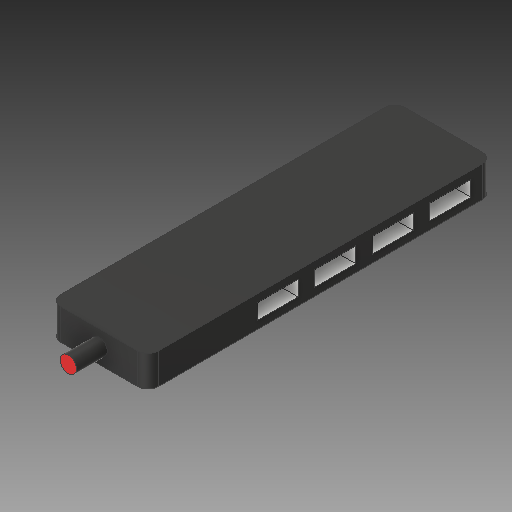
# Autodesk Inventor part: usbHub
Saved by Autodesk Inventor 2018 (Build 220112000, 112)
## iProperties
Created: 2018-08-03
Part Number: usbHub
Material: ABS Plastic
Document SubType Name: Modeling
Designer: Cole Tucker
Density: 1.06 g/cm^3
Appearance: Smooth - White
Mass: 30.4132 g
Surface Area: 110.112 cm^2
Volume: 28.6917 cm^3
Author: Cole Tucker
Autodesk Inventor part; units mm, degrees
ref_plane "YZ Plane" through (0, 0, 0) normal (1, 0, 0) x (0, 1, 0)
ref_plane "XZ Plane" through (0, 0, 0) normal (0, 1, 0) x (-1, 0, 0)
ref_plane "XY Plane" through (0, 0, 0) normal (0, 0, 1) x (1, 0, 0)
sketch "Sketch1" plane through (0, 0, 0) normal (0, 1, 0) x (-1, 0, 0)
  line L0 (0, 0) -> (30.1625, 0)
  line L1 (30.1625, 0) -> (30.1625, -106.3625)
  line L2 (30.1625, -106.3625) -> (0, -106.3625)
  line L3 (0, -106.3625) -> (0, 0)
  dimension "d0" = 30.1625
  dimension "d1" = 106.3625
  constraints: 8 end point, 2 parallel, 1 horizontal, 1 perpendicular
  measures "d0" distance of L1.end L2.end
  measures "d1" distance of L0.end L1.end
extrude "Extrusion1" add sketch "Sketch1" along normal blind 9.525
sketch "Sketch2" plane through (0, 0, 0) normal (1, 0, 0) x (0, 0, -1)
  line L0 (0, 0) -> (0, 9.525) construction
  line L1 (0, 9.525) -> (106.3625, 9.525) construction
  line L2 (106.3625, 0) -> (106.3625, 9.525) construction
  line L3 (28.575, 9.525) -> (106.3625, 9.525) construction
  line L4 (106.3625, 9.525) -> (106.3625, 0) construction
  line L5 (106.3625, 0) -> (28.575, 0) construction
  line L6 (28.575, 0) -> (28.575, 9.525) construction
  line L7 (28.575, 4.7625) -> (28.575, 0) construction
  line L8 (28.575, 4.7625) -> (28.575, 2.3813) construction
  line L9 (28.575, 2.3813) -> (33.655, 2.3813) construction
  line L10 (33.655, 2.3813) -> (46.355, 2.3813)
  line L11 (46.355, 2.3813) -> (46.355, 7.1437)
  line L12 (46.355, 7.1437) -> (33.655, 7.1438)
  line L13 (33.655, 7.1438) -> (33.655, 2.3813)
  line L14 (46.355, 2.3813) -> (51.435, 2.3813) construction
  line L15 (51.435, 2.3813) -> (64.135, 2.3813)
  line L16 (64.135, 2.3813) -> (64.135, 7.1437)
  line L17 (64.135, 7.1437) -> (51.435, 7.1437)
  line L18 (51.435, 7.1437) -> (51.435, 2.3813)
  line L19 (64.135, 2.3813) -> (69.215, 2.3813)
  line L20 (69.215, 2.3813) -> (81.915, 2.3813)
  line L21 (81.915, 2.3813) -> (81.915, 7.1437)
  line L22 (81.915, 7.1437) -> (69.215, 7.1437)
  line L23 (69.215, 7.1437) -> (69.215, 2.3813)
  line L24 (81.915, 2.3813) -> (86.995, 2.3813)
  line L25 (81.915, 7.1437) -> (81.915, 2.3813)
  line L26 (86.995, 2.3813) -> (99.695, 2.3813)
  line L27 (99.695, 2.3813) -> (99.695, 7.1437)
  line L28 (99.695, 7.1437) -> (86.995, 7.1437)
  line L29 (86.995, 7.1437) -> (86.995, 2.3813)
  dimension "d7" = 2.3813
  dimension "d9" = 12.7
  dimension "d10" = 4.7625
  dimension "d12" = 12.7
  dimension "d13" = 4.7625
  dimension "d15" = 12.7
  dimension "d16" = 4.7625
  dimension "d20" = 28.575
  dimension "d21" = 12.7
  dimension "d22" = 4.7625
  dimension "d23" = 5.08
  dimension "d24" = 5.08
  dimension "d25" = 5.08
  dimension "d26" = 5.08
  constraints: 54 end point, 10 parallel, 9 horizontal, 5 perpendicular, 1 collinear, 1 midpoint, 1 point on line
  measures "d7" distance of L7.start L8.end
  measures "d9" distance of L12.end L11.end
  measures "d10" distance of L11.end L10.end
  measures "d12" distance of L17.end L16.end
  measures "d13" distance of L16.end L15.end
  measures "d15" distance of L22.end L21.end
  measures "d16" distance of L21.end L20.end
  measures "d20" distance between parallel lines of L0 L6
  measures "d21" distance of L28.end L27.end
  measures "d22" distance of L27.end L26.end
  measures "d23" distance of L20.end L24.end
  measures "d24" distance between parallel lines of L6 L13
  measures "d25" distance of L10.end L14.end
  measures "d26" distance of L15.end L19.end
extrude "Extrusion2" cut sketch "Sketch2" against normal blind 9.525
fillet "Fillet1" radius 3.175 4 edges at (0, 4.7625, 0) (-30.1625, 4.7625, 0) (-30.1625, 4.7625, -106.3625) (0, 4.7625, -106.3625)
sketch "Sketch3" plane through (-26.9875, 0, 0) normal (0, 0, 1) x (1, 0, 0)
  line L0 (0, 0) -> (23.8125, 0) construction
  line L1 (11.9062, 0) -> (11.9062, 9.525) construction
  line L2 (23.8125, 9.525) -> (0, 9.525) construction
  circle A0 centre (11.9062, 4.7625) radius 2.54
  point P0 (26.9875, 0)
  dimension "d30" = 5.08
  constraints: 3 midpoint, 2 end point, 1 centre point
  measures "d30" diameter of A0
extrude "Extrusion3" add sketch "Sketch3" along normal blind 9.525
sketch "Sketch4" plane through (-9.525, 0, 0) normal (1, 0, 0) x (0, 0, -1)
  line L0 (33.655, 2.3813) -> (33.655, 7.1438) construction
  line L1 (33.655, 4.7625) -> (99.695, 4.7625) construction
  line L2 (99.695, 7.1437) -> (99.695, 2.3813) construction
  line L3 (40.005, 4.7625) -> (34.925, 4.7625) construction
  line L4 (34.925, 4.7625) -> (34.925, 6.0325) construction
  line L5 (34.925, 6.0325) -> (40.005, 6.0325) construction
  line L6 (40.005, 6.0325) -> (40.005, 4.7625) construction
  line L7 (57.785, 4.7625) -> (52.705, 4.7625) construction
  line L8 (52.705, 4.7625) -> (52.705, 6.0325) construction
  line L9 (52.705, 6.0325) -> (57.785, 6.0325) construction
  line L10 (57.785, 6.0325) -> (57.785, 4.7625) construction
  line L11 (75.565, 4.7625) -> (70.485, 4.7625) construction
  line L12 (70.485, 4.7625) -> (70.485, 6.0325) construction
  line L13 (70.485, 6.0325) -> (75.565, 6.0325) construction
  line L14 (75.565, 6.0325) -> (75.565, 4.7625) construction
  line L15 (93.345, 4.7625) -> (88.265, 4.7625) construction
  line L16 (88.265, 4.7625) -> (88.265, 6.0325) construction
  line L17 (88.265, 6.0325) -> (93.345, 6.0325) construction
  line L18 (93.345, 6.0325) -> (93.345, 4.7625) construction
  line L19 (93.345, 4.7625) -> (98.425, 4.7625) construction
  line L20 (75.565, 4.7625) -> (80.645, 4.7625) construction
  line L21 (57.785, 4.7625) -> (62.865, 4.7625) construction
  line L22 (40.005, 4.7625) -> (45.085, 4.7625) construction
  line L23 (34.925, 6.0325) -> (45.085, 6.0325)
  line L24 (45.085, 6.0325) -> (45.085, 4.7625)
  line L25 (45.085, 4.7625) -> (34.925, 4.7625)
  line L26 (34.925, 4.7625) -> (34.925, 6.0325)
  line L27 (52.705, 6.0325) -> (62.865, 6.0325)
  line L28 (62.865, 6.0325) -> (62.865, 4.7625)
  line L29 (62.865, 4.7625) -> (52.705, 4.7625)
  line L30 (52.705, 4.7625) -> (52.705, 6.0325)
  line L31 (70.485, 6.0325) -> (80.645, 6.0325)
  line L32 (80.645, 6.0325) -> (80.645, 4.7625)
  line L33 (80.645, 4.7625) -> (70.485, 4.7625)
  line L34 (70.485, 4.7625) -> (70.485, 6.0325)
  line L35 (88.265, 6.0325) -> (98.425, 6.0325)
  line L36 (98.425, 6.0325) -> (98.425, 4.7625)
  line L37 (98.425, 4.7625) -> (88.265, 4.7625)
  line L38 (88.265, 4.7625) -> (88.265, 6.0325)
  point P0 (0, 0)
  dimension "d33" = 5.08
  dimension "d34" = 1.27
  dimension "d35" = 5.08
  dimension "d36" = 1.27
  dimension "d37" = 5.08
  dimension "d38" = 1.27
  dimension "d39" = 5.08
  dimension "d40" = 1.27
  dimension "d41" = 5.08
  dimension "d42" = 5.08
  dimension "d43" = 5.08
  dimension "d44" = 5.08
  constraints: 72 end point, 16 parallel, 8 horizontal, 8 perpendicular, 2 midpoint, 11 other
  measures "d33" distance of L4.end L5.end
  measures "d34" distance of L3.end L4.end
  measures "d35" distance of L8.end L9.end
  measures "d36" distance of L7.end L8.end
  measures "d37" distance of L12.end L13.end
  measures "d38" distance of L11.end L12.end
  measures "d39" distance of L16.end L17.end
  measures "d40" distance of L15.end L16.end
  measures "d41" distance of L15.start L19.end
  measures "d42" distance of L11.start L20.end
  measures "d43" distance of L7.start L21.end
  measures "d44" distance of L3.start L22.end
extrude "Extrusion4" add sketch "Sketch4" along normal blind 6.35
body "Solid1"
